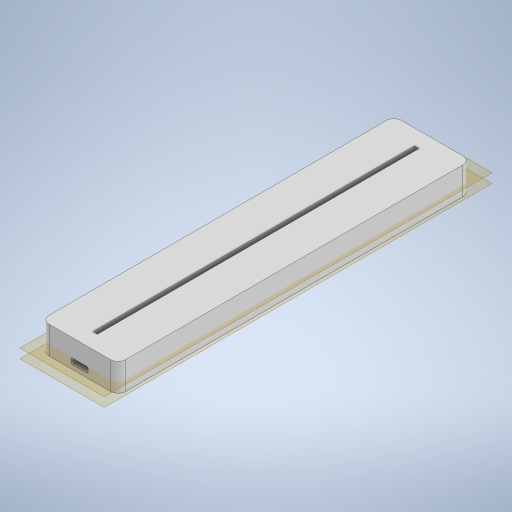
# Autodesk Inventor part: acrylic_base
Saved by Autodesk Inventor 2024 (Build 280153000, 153)
## iProperties
Created: 2023-06-28
Part Number: acrylic_base
Material: Generic
Document SubType Name: Modeling
Designer: LabTel_Admin
Density: 1 g/cm^3
Appearance: Default
Author: LabTel_Admin
Autodesk Inventor part; units mm, degrees
ref_plane "YZ Plane" through (0, 0, 0) normal (1, 0, 0) x (0, 1, 0)
ref_plane "XZ Plane" through (0, 0, 0) normal (0, 1, 0) x (-1, 0, 0)
ref_plane "XY Plane" through (0, 0, 0) normal (0, 0, 1) x (1, 0, 0)
sketch "Sketch1" plane through (0, 0, 0) normal (0, 1, 0) x (-1, 0, 0)
  line L0 (-20, -115) -> (20, -115)
  line L1 (25, -110) -> (25, 110)
  line L2 (20, 115) -> (-20, 115)
  line L3 (-25, 110) -> (-25, -110)
  line L4 (-5, -105) -> (5, -105)
  line L5 (5, -105) -> (5, 105)
  line L6 (5, 105) -> (-5, 105)
  line L7 (-5, 105) -> (-5, -105)
  arc A0 (25, 110) -> (20, 115) centre (20, 110) ccw
  arc A1 (-20, 115) -> (-25, 110) centre (-20, 110) ccw
  arc A2 (-25, -110) -> (-20, -115) centre (-20, -110) ccw
  arc A3 (20, -115) -> (25, -110) centre (20, -110) ccw
  line L8 (-1.5, -105) -> (1.5, -105)
  line L9 (1.5, 105) -> (-1.5, 105)
  point P0 (0, 0)
  point P1 (0, 0)
  dimension "d6" = 10
  dimension "d7" = 210
  dimension "d8" = 5
  dimension "d9" = 3
  dimension "d10" = 210
  constraints: 20 end point, 8 point on circle, 8 tangent, 5 parallel, 4 centre point, 3 equal radius, 3 horizontal, 2 perpendicular
  measures "d6" distance of L6.end L5.end
  measures "d7" distance of L5.end L4.end
  measures "d8" radius of A0
  measures "d9" distance of L9.end L9.start
  measures "d10" distance of L9.start L8.end
extrude "Extrusion1" add sketch "Sketch1" along normal blind 30
extrude "Extrusion2" add sketch "Sketch1" along normal blind 15 contours L7 L6 L5 L4
sketch "Sketch2" plane through (0, 30, 0) normal (0, 1, 0) x (1, 0, 0)
  line L0 (-1.5, -105) -> (1.5, -105)
  line L1 (1.5, -105) -> (1.5, 105)
  line L2 (1.5, 105) -> (-1.5, 105)
  line L3 (-1.5, 105) -> (-1.5, -105)
  line L4 (-1.5, -105) -> (1.5, 105) construction
  line L5 (1.5, -105) -> (-1.5, 105) construction
  line L6 (5, 105) -> (5, -105) projected
  line L7 (5, 105) -> (1.5, 105)
  line L8 (1.5, 105) -> (1.5, -105)
  line L9 (1.5, -105) -> (5, -105)
  line L10 (5, -105) -> (5, 105)
  line L11 (-5, 105) -> (5, 105) projected
  line L12 (-5, 105) -> (-1.5, 105)
  line L13 (-1.5, 105) -> (-1.5, -105)
  line L14 (-1.5, -105) -> (-5, -105)
  line L15 (-5, -105) -> (-5, 105)
  point P0 (0, 0)
  dimension "d15" = 3
  dimension "d16" = 210
  constraints: 28 end point, 6 parallel, 3 horizontal, 3 perpendicular, 2 midpoint
  measures "d15" distance of L2.end L1.end
  measures "d16" distance of L1.end L0.end
extrude "Extrusion3" add sketch "Sketch2" against normal blind 15 contours L14 L15 L11 L3 | L1 L7 L6 L9
sketch "Sketch5" plane through (-20, 0, 115) normal (0, 0, 1) x (1, 0, 0)
  line L0 (15.5, 15) -> (24.5, 15)
  line L1 (25.5, 16) -> (25.5, 17.5)
  line L2 (24.5, 18.5) -> (15.5, 18.5)
  line L3 (14.5, 17.5) -> (14.5, 16)
  arc A0 (15.5, 18.5) -> (14.5, 17.5) centre (15.5, 17.5) ccw
  arc A1 (14.5, 16) -> (15.5, 15) centre (15.5, 16) ccw
  arc A2 (24.5, 15) -> (25.5, 16) centre (24.5, 16) ccw
  arc A3 (25.5, 17.5) -> (24.5, 18.5) centre (24.5, 17.5) ccw
  line L4 (-5, 0) -> (-5, 30) projected
  point P0 (20, 0)
  point P1 (14.5, 15)
  point P2 (25.5, 18.5)
  point P3 (25.5, 15)
  point P4 (14.5, 18.5)
  point P5 (14.5, 16.75)
  dimension "d23" = 11
  dimension "d24" = 3.5
  dimension "d27" = 1
  dimension "d38" = 19.5
  constraints: 8 end point, 8 point on circle, 8 point on line, 8 tangent, 4 centre point, 3 equal radius, 2 parallel, 1 horizontal, 1 midpoint, 1 perpendicular
  measures "d23" distance of point (14.5, 18.5) point (25.5, 18.5)
  measures "d24" distance of point (25.5, 18.5) point (25.5, 15)
  measures "d27" radius of A0
  measures "d38" distance from line of L4 point (14.5, 16.75)
extrude "Extrusion4" cut sketch "Sketch5" against normal blind 225
ref_plane "Work Plane1" through (0, 18.5, 0) normal (0, 1, 0) x (1, 0, 0)
sketch "Sketch6" plane through (0, 18.5, 0) normal (0, 1, 0) x (1, 0, 0)
  line L0 (-1.5, -105) -> (1.5, -105)
  line L1 (1.5, -105) -> (1.5, -101.5)
  line L2 (1.5, -101.5) -> (-1.5, -101.5)
  line L3 (-1.5, -101.5) -> (-1.5, -105)
  line L4 (0, 0) -> (38.1374, 0)
  line L5 (-1.5, 105) -> (1.5, 105)
  line L6 (1.5, 105) -> (1.5, 101.5)
  line L7 (1.5, 101.5) -> (-1.5, 101.5)
  line L8 (-1.5, 101.5) -> (-1.5, 105)
  dimension "d31" = 3.5
  constraints: 18 end point, 4 symmetric about line, 2 horizontal, 2 parallel, 1 perpendicular
  measures "d31" distance of L1.end L0.end
extrude "Extrusion5" add sketch "Sketch6" along normal blind 4.5
ref_plane "Work Plane2" through (0, 12.5, 0) normal (0, 1, 0) x (1, 0, 0)
move faces "Move1" translate (0, 12, 0) faces at (8.3333, 0, 36.6667)
body "Solid1"
